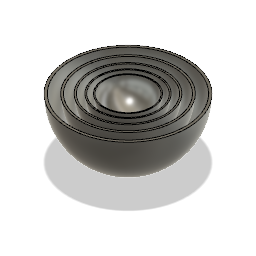
rolling ball v1 (Autodesk Fusion 360 design; units mm, degrees)
Autodesk Fusion 360 part; units mm, degrees
note: some values were not read from the file. Chosen so that the rebuilt part matches the saved one: which bodies a step acts on.
sphere "SpherePrimitive1" add diameter 120 placed x (1, 0, 0) y (0, 1, 0) z (0, 0, 1) at (0, 0, 0) makes body 1
shell "Shell1" thickness 2.5 removed faces 0 bodies 1
split "Split1" by plane through (0, 0, 0) normal (0, 1, 0) bodies 1 makes body 2 at (56.8845, 14.1829, -12.7672)
delete_body "RemoveBody1" bodies 2
copy_body "CopyPasteBodies1" bodies 1 makes body 3
scale "Scale1" factor 0.8 about (0, 0, 0) bodies 3
copy_body "CopyPasteBodies2" bodies 3 makes body 4
scale "Scale2" factor 0.8 about (0, 0, 0) bodies 4
copy_body "CopyPasteBodies3" bodies 4 makes body 5
scale "Scale3" factor 0.8 about (0, 0, 0) bodies 5
copy_body "CopyPasteBodies4" bodies 5 makes body 6
scale "Scale4" factor 0.8 about (0, 0, 0) bodies 6
copy_body "Body->Comp1" bodies 1 removing the originals makes body 7 in component "Component"
copy_body "Body->Comp2" bodies 3 removing the originals makes body 8 in component "Component'"
copy_body "Body->Comp3" bodies 4 removing the originals makes body 9 in component "Component''"
copy_body "Body->Comp4" bodies 5 removing the originals makes body 10 in component "Component'''"
copy_body "Body->Comp5" bodies 6 removing the originals makes body 11 in component "Component''''"
component "Component" placed x (1, 0, 0) y (0, 1, 0) z (0, 0, 1) at (0, 0, 0)
component "Component'" placed x (1, 0, 0) y (0, 1, 0) z (0, 0, 1) at (0, 0, 0)
component "Component''" placed x (1, 0, 0) y (0, 1, 0) z (0, 0, 1) at (0, 0, 0)
component "Component'''" placed x (1, 0, 0) y (0, 1, 0) z (0, 0, 1) at (0, 0, 0)
component "Component''''" placed x (1, 0, 0) y (0, 1, 0) z (0, 0, 1) at (0, 0, 0)
